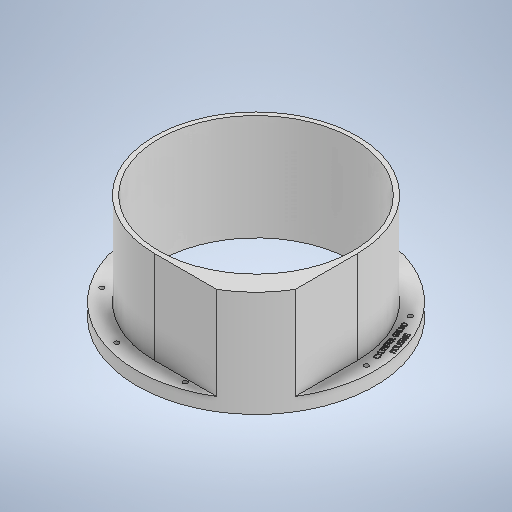
# Autodesk Inventor part: Cylinder Housing
Saved by Autodesk Inventor 2025 (Build 290162000, 162)
## iProperties
Created: 2025-06-17
Part Number: Cylinder Housing
Material: Generic
Document SubType Name: Modeling
Designer: mumin
Density: 1 g/cm^3
Appearance: Default
Author: mumin
Autodesk Inventor part; units mm, degrees
ref_plane "YZ Plane" through (0, 0, 0) normal (1, 0, 0) x (0, 1, 0)
ref_plane "XZ Plane" through (0, 0, 0) normal (0, 1, 0) x (-1, 0, 0)
ref_plane "XY Plane" through (0, 0, 0) normal (0, 0, 1) x (1, 0, 0)
sketch "Sketch1" plane through (0, 0, 0) normal (0, 1, 0) x (-1, 0, 0)
  circle A0 centre (0, 0) radius 110
  circle A1 centre (0, 0) radius 135
  dimension "d0" = 220
  dimension "d1" = 270
  constraints: 2 centre point, 2 coincident
  measures "d0" diameter of A0
  measures "d1" diameter of A1
extrude "Extrusion1" add sketch "Sketch1" along normal blind 15
sketch "Sketch5" plane through (0, 15, 0) normal (0, 1, 0) x (1, 0, 0)
  line L0 (-189, 0) -> (189, 0) projected
  point P0 (0, 0)
  point P1 (-125, 0)
  dimension "d23" = 125
  constraints: 1 point on line
  measures "d23" distance of point (0, 0) point (-125, 0)
hole "Hole2" at (-125, 15, 0) direction (0, -1, 0) diameter 5.2 end through all
pattern_circular "Circular Pattern1" count 10 over 360 about axis through (0, -10, 0) along (0, 1, 0) of "Hole2"
sketch "Sketch6" plane through (0, 0, 0) normal (0, 1, 0) x (-1, 0, 0)
  circle A0 centre (0, 0) radius 110 projected
  circle A1 centre (0, 0) radius 135 projected
  circle A2 centre (0, 0) radius 115
  line L0 (0, 115) -> (-115, 115)
  line L1 (-115, 115) -> (-115, 0)
  point P0 (-70.7107, 115)
  point P1 (-115, 70.7107)
  dimension "d27" = 230
  constraints: 4 end point, 2 point on circle, 2 tangent, 1 centre point, 1 coincident, 1 horizontal
  measures "d27" diameter of A2
extrude "Extrusion4" add sketch "Sketch6" along normal blind 120 contours L0 A2 L1 A1 | A2 picked at (-94.2438, 86.8114)
sketch "Sketch7" plane through (0, 15, 0) normal (0, 1, 0) x (1, 0, 0)
  line L0 (121.4652, 9.1206) -> (102.4195, 65.4859) construction
  line L1 (102.4195, 65.4859) -> (106.7219, 66.9397) construction
  line L2 (106.7219, 66.9397) -> (125.7676, 10.5743) construction
  line L3 (125.7676, 10.5743) -> (121.4652, 9.1206) construction
  spline S0 degree 2 poles (124.8327, 15.3814) (124.9884, 14.9208) (124.9407, 14.0365) (124.7258, 13.6474) knots 0 0 0 1 2 2 2
  spline S1 degree 2 poles (124.7258, 13.6474) (124.5147, 13.2596) (123.6985, 12.6373) (123.0996, 12.435) knots 0 0 0 1 2 2 2
  spline S2 degree 2 poles (123.0996, 12.435) (122.5046, 12.2339) (121.5193, 12.2389) (121.0957, 12.4165) knots 0 0 0 1 2 2 2
  spline S3 degree 2 poles (121.0957, 12.4165) (120.6811, 12.5929) (120.0852, 13.2555) (119.923, 13.7353) knots 0 0 0 1 2 2 2
  spline S4 degree 2 poles (119.923, 13.7353) (119.8426, 13.9733) (119.7703, 14.4151) (119.7644, 14.6098) knots 0 0 0 1 2 2 2
  spline S5 degree 2 poles (119.7644, 14.6098) (119.7624, 14.7802) (119.7968, 15.1468) (119.8281, 15.3327) knots 0 0 0 1 2 2 2
  line L4 (119.8281, 15.3327) -> (120.5881, 15.5895)
  line L5 (120.5881, 15.5895) -> (120.605, 15.5396)
  spline S6 degree 2 poles (120.605, 15.5396) (120.5567, 15.4293) (120.43, 15.0956) (120.3899, 14.8725) knots 0 0 0 1 2 2 2
  spline S7 degree 2 poles (120.3899, 14.8725) (120.351, 14.6583) (120.3683, 14.1894) (120.4617, 13.9131) knots 0 0 0 1 2 2 2
  spline S8 degree 2 poles (120.4617, 13.9131) (120.5642, 13.6098) (120.9966, 13.1529) (121.3033, 13.0298) knots 0 0 0 1 2 2 2
  spline S9 degree 2 poles (121.3033, 13.0298) (121.6126, 12.9119) (122.421, 12.937) (122.8778, 13.0914) knots 0 0 0 1 2 2 2
  spline S10 degree 2 poles (122.8778, 13.0914) (123.3653, 13.2561) (123.9887, 13.7276) (124.1618, 14.0128) knots 0 0 0 1 2 2 2
  spline S11 degree 2 poles (124.1618, 14.0128) (124.3285, 14.2915) (124.3862, 14.9055) (124.285, 15.2049) knots 0 0 0 1 2 2 2
  spline S12 degree 2 poles (124.285, 15.2049) (124.1929, 15.4775) (123.9016, 15.8966) (123.7409, 16.0433) knots 0 0 0 1 2 2 2
  spline S13 degree 2 poles (123.7409, 16.0433) (123.5827, 16.1823) (123.2885, 16.3694) (123.1909, 16.4177) knots 0 0 0 1 2 2 2
  line L6 (123.1909, 16.4177) -> (123.1754, 16.4638)
  line L7 (123.1754, 16.4638) -> (123.9277, 16.718)
  spline S14 degree 2 poles (123.9277, 16.718) (124.0539, 16.5853) (124.2816, 16.3543) (124.4092, 16.1793) knots 0 0 0 1 2 2 2
  spline S15 degree 2 poles (124.4092, 16.1793) (124.5483, 15.9953) (124.7367, 15.6655) (124.8327, 15.3814) knots 0 0 0 1 2 2 2
  line L8 (118.1942, 19.1303) -> (121.376, 18.4219)
  line L9 (121.376, 18.4219) -> (123.4719, 19.1301)
  line L10 (123.4719, 19.1301) -> (123.6847, 18.5006)
  line L11 (123.6847, 18.5006) -> (121.654, 17.8145)
  line L12 (121.654, 17.8145) -> (119.4887, 15.2993)
  line L13 (119.4887, 15.2993) -> (119.2526, 15.9979)
  line L14 (119.2526, 15.9979) -> (120.9232, 17.9268)
  line L15 (120.9232, 17.9268) -> (118.4199, 18.4623)
  line L16 (118.4199, 18.4623) -> (118.1942, 19.1303)
  line L17 (121.8558, 23.9131) -> (122.7832, 21.1685)
  line L18 (122.7832, 21.1685) -> (118.0463, 19.5679)
  line L19 (118.0463, 19.5679) -> (117.8336, 20.1974)
  line L20 (117.8336, 20.1974) -> (122.01, 21.6086)
  line L21 (122.01, 21.6086) -> (121.2954, 23.7237)
  line L22 (121.2954, 23.7237) -> (121.8558, 23.9131)
  line L23 (121.1307, 26.0589) -> (121.7507, 24.224)
  line L24 (121.7507, 24.224) -> (121.2671, 24.0606)
  line L25 (121.2671, 24.0606) -> (121.0634, 24.6633)
  line L26 (121.0634, 24.6633) -> (117.2939, 23.3895)
  line L27 (117.2939, 23.3895) -> (117.4975, 22.7869)
  line L28 (117.4975, 22.7869) -> (117.0138, 22.6234)
  line L29 (117.0138, 22.6234) -> (116.3938, 24.4583)
  line L30 (116.3938, 24.4583) -> (116.8775, 24.6217)
  line L31 (116.8775, 24.6217) -> (117.0812, 24.0191)
  line L32 (117.0812, 24.0191) -> (120.8507, 25.2928)
  line L33 (120.8507, 25.2928) -> (120.6471, 25.8955)
  line L34 (120.6471, 25.8955) -> (121.1307, 26.0589)
  line L35 (119.7221, 30.2277) -> (119.9608, 29.5214)
  line L36 (119.9608, 29.5214) -> (116.5847, 26.0454)
  line L37 (116.5847, 26.0454) -> (120.669, 27.4255)
  line L38 (120.669, 27.4255) -> (120.8674, 26.8381)
  line L39 (120.8674, 26.8381) -> (116.1305, 25.2376)
  line L40 (116.1305, 25.2376) -> (115.8283, 26.132)
  line L41 (115.8283, 26.132) -> (118.934, 29.307)
  line L42 (118.934, 29.307) -> (115.1837, 28.0398)
  line L43 (115.1837, 28.0398) -> (114.9852, 28.6271)
  line L44 (114.9852, 28.6271) -> (119.7221, 30.2277)
  spline S16 degree 2 poles (115.7712, 34.1233) (116.4199, 34.3425) (117.6417, 34.1695) (118.0826, 33.8266) knots 0 0 0 1 2 2 2
  spline S17 degree 2 poles (118.0826, 33.8266) (118.431, 33.5423) (118.8349, 32.8533) (119.0295, 32.2775) knots 0 0 0 1 2 2 2
  line L45 (119.0295, 32.2775) -> (119.3978, 31.1873)
  line L46 (119.3978, 31.1873) -> (114.661, 29.5867)
  line L47 (114.661, 29.5867) -> (114.2965, 30.6654)
  spline S18 degree 2 poles (114.2965, 30.6654) (114.0708, 31.3333) (114.0136, 32.1608) (114.0994, 32.4892) knots 0 0 0 1 2 2 2
  spline S19 degree 2 poles (114.0994, 32.4892) (114.2483, 33.0485) (115.0802, 33.8899) (115.7712, 34.1233) knots 0 0 0 1 2 2 2
  spline S20 degree 2 poles (115.9853, 33.4643) (115.4402, 33.2802) (114.7906, 32.6586) (114.6924, 32.2277) knots 0 0 0 1 2 2 2
  spline S21 degree 2 poles (114.6924, 32.2277) (114.6283, 31.9237) (114.6872, 31.3064) (114.8312, 30.8803) knots 0 0 0 1 2 2 2
  line L48 (114.8312, 30.8803) -> (114.9933, 30.4005)
  line L49 (114.9933, 30.4005) -> (118.64, 31.6327)
  line L50 (118.64, 31.6327) -> (118.4779, 32.1125)
  spline S22 degree 2 poles (118.4779, 32.1125) (118.3365, 32.5309) (117.9882, 33.1189) (117.7208, 33.3151) knots 0 0 0 1 2 2 2
  spline S23 degree 2 poles (117.7208, 33.3151) (117.3866, 33.57) (116.5381, 33.6511) (115.9853, 33.4643) knots 0 0 0 1 2 2 2
  line L51 (117.9049, 35.6056) -> (113.168, 34.005)
  line L52 (113.168, 34.005) -> (112.1667, 36.9685)
  line L53 (112.1667, 36.9685) -> (112.7271, 37.1578)
  line L54 (112.7271, 37.1578) -> (113.5158, 34.8239)
  line L55 (113.5158, 34.8239) -> (114.8132, 35.2623)
  line L56 (114.8132, 35.2623) -> (114.0778, 37.4389)
  line L57 (114.0778, 37.4389) -> (114.6382, 37.6282)
  line L58 (114.6382, 37.6282) -> (115.3737, 35.4517)
  line L59 (115.3737, 35.4517) -> (117.1318, 36.0458)
  line L60 (117.1318, 36.0458) -> (116.3431, 38.3797)
  line L61 (116.3431, 38.3797) -> (116.9036, 38.569)
  line L62 (116.9036, 38.569) -> (117.9049, 35.6056)
  line L63 (115.4314, 42.9259) -> (115.7077, 42.1083)
  line L64 (115.7077, 42.1083) -> (114.3288, 39.9743)
  line L65 (114.3288, 39.9743) -> (114.5726, 39.2527)
  line L66 (114.5726, 39.2527) -> (116.4574, 39.8895)
  line L67 (116.4574, 39.8895) -> (116.6701, 39.26)
  line L68 (116.6701, 39.26) -> (111.9332, 37.6594)
  line L69 (111.9332, 37.6594) -> (111.5207, 38.8801)
  spline S24 degree 2 poles (111.5207, 38.8801) (111.3833, 39.287) (111.2861, 39.8658) (111.363, 40.1698) knots 0 0 0 1 2 2 2
  spline S25 degree 2 poles (111.363, 40.1698) (111.4399, 40.4737) (111.8455, 40.9316) (112.2178, 41.0574) knots 0 0 0 1 2 2 2
  spline S26 degree 2 poles (112.2178, 41.0574) (112.736, 41.2325) (113.6175, 40.9401) (113.9395, 40.5442) knots 0 0 0 1 2 2 2
  line L70 (113.9395, 40.5442) -> (115.4314, 42.9259)
  spline S27 degree 2 poles (112.4895, 40.4178) (112.2822, 40.3478) (112.0129, 40.0943) (111.9612, 39.9057) knots 0 0 0 1 2 2 2
  spline S28 degree 2 poles (111.9612, 39.9057) (111.9183, 39.7415) (111.966, 39.3599) (112.0542, 39.0988) knots 0 0 0 1 2 2 2
  line L71 (112.0542, 39.0988) -> (112.2656, 38.4731)
  line L72 (112.2656, 38.4731) -> (114.0467, 39.075)
  line L73 (114.0467, 39.075) -> (113.8599, 39.6277)
  spline S29 degree 2 poles (113.8599, 39.6277) (113.7678, 39.9003) (113.5253, 40.3016) (113.325, 40.4008) knots 0 0 0 1 2 2 2
  spline S30 degree 2 poles (113.325, 40.4008) (113.1478, 40.4948) (112.7352, 40.5008) (112.4895, 40.4178) knots 0 0 0 1 2 2 2
  spline S31 degree 2 poles (114.0384, 47.3523) (114.2083, 46.8494) (114.1827, 45.9127) (113.9729, 45.5082) knots 0 0 0 1 2 2 2
  spline S32 degree 2 poles (113.9729, 45.5082) (113.7593, 45.1024) (112.938, 44.4699) (112.3354, 44.2663) knots 0 0 0 1 2 2 2
  spline S33 degree 2 poles (112.3354, 44.2663) (111.7634, 44.073) (110.7485, 44.0894) (110.3249, 44.2798) knots 0 0 0 1 2 2 2
  spline S34 degree 2 poles (110.3249, 44.2798) (109.9167, 44.4627) (109.2935, 45.193) (109.1236, 45.6959) knots 0 0 0 1 2 2 2
  spline S35 degree 2 poles (109.1236, 45.6959) (109.0419, 45.9377) (108.9631, 46.3987) (108.9571, 46.619) knots 0 0 0 1 2 2 2
  spline S36 degree 2 poles (108.9571, 46.619) (108.9487, 46.7958) (108.9853, 47.2444) (109.0065, 47.3842) knots 0 0 0 1 2 2 2
  line L74 (109.0065, 47.3842) -> (109.7666, 47.641)
  line L75 (109.7666, 47.641) -> (109.7847, 47.5873)
  spline S37 degree 2 poles (109.7847, 47.5873) (109.7213, 47.4332) (109.6175, 47.1202) (109.5878, 46.8535) knots 0 0 0 1 2 2 2
  spline S38 degree 2 poles (109.5878, 46.8535) (109.5567, 46.6292) (109.5974, 46.0912) (109.6934, 45.8071) knots 0 0 0 1 2 2 2
  spline S39 degree 2 poles (109.6934, 45.8071) (109.9242, 45.1239) (111.2383, 44.627) (112.0944, 44.9162) knots 0 0 0 1 2 2 2
  spline S40 degree 2 poles (112.0944, 44.9162) (112.5704, 45.077) (113.2091, 45.5409) (113.3834, 45.8351) knots 0 0 0 1 2 2 2
  spline S41 degree 2 poles (113.3834, 45.8351) (113.5604, 46.1215) (113.623, 46.7842) (113.5011, 47.1451) knots 0 0 0 1 2 2 2
  spline S42 degree 2 poles (113.5011, 47.1451) (113.4116, 47.4099) (113.1558, 47.9137) (113.0181, 48.0682) knots 0 0 0 1 2 2 2
  line L76 (113.0181, 48.0682) -> (111.7936, 47.6544)
  line L77 (111.7936, 47.6544) -> (112.1645, 46.5566)
  line L78 (112.1645, 46.5566) -> (111.6117, 46.3698)
  line L79 (111.6117, 46.3698) -> (111.0307, 48.0895)
  line L80 (111.0307, 48.0895) -> (113.0997, 48.7886)
  spline S43 degree 2 poles (113.0997, 48.7886) (113.1936, 48.6878) (113.4962, 48.3367) (113.6045, 48.1808) knots 0 0 0 1 2 2 2
  spline S44 degree 2 poles (113.6045, 48.1808) (113.7527, 47.97) (113.9489, 47.6172) (114.0384, 47.3523) knots 0 0 0 1 2 2 2
  line L81 (113.3198, 49.1752) -> (108.0433, 49.1715)
  line L82 (108.0433, 49.1715) -> (107.7813, 49.9469)
  line L83 (107.7813, 49.9469) -> (111.9786, 53.1444)
  line L84 (111.9786, 53.1444) -> (112.203, 52.4803)
  line L85 (112.203, 52.4803) -> (111.0239, 51.6029)
  line L86 (111.0239, 51.6029) -> (111.6349, 49.7949)
  line L87 (111.6349, 49.7949) -> (113.1045, 49.8124)
  line L88 (113.1045, 49.8124) -> (113.3198, 49.1752)
  line L89 (110.5449, 51.2486) -> (108.5624, 49.7618)
  line L90 (108.5624, 49.7618) -> (111.0391, 49.786)
  line L91 (111.0391, 49.786) -> (110.5449, 51.2486)
  line L92 (110.8994, 56.3381) -> (111.8268, 53.5935)
  line L93 (111.8268, 53.5935) -> (107.09, 51.9929)
  line L94 (107.09, 51.9929) -> (106.8772, 52.6225)
  line L95 (106.8772, 52.6225) -> (111.0537, 54.0337)
  line L96 (111.0537, 54.0337) -> (110.339, 56.1488)
  line L97 (110.339, 56.1488) -> (110.8994, 56.3381)
  line L98 (104.8344, 58.6683) -> (110.1225, 58.6375)
  line L99 (110.1225, 58.6375) -> (110.3521, 57.9581)
  line L100 (110.3521, 57.9581) -> (106.1664, 54.726)
  line L101 (106.1664, 54.726) -> (105.9382, 55.4016)
  line L102 (105.9382, 55.4016) -> (109.4292, 58.044)
  line L103 (109.4292, 58.044) -> (105.051, 58.0273)
  line L104 (105.051, 58.0273) -> (104.8344, 58.6683)
  spline S45 degree 2 poles (104.0902, 62.6553) (104.3142, 63.0304) (105.1343, 63.6411) (105.7254, 63.8408) knots 0 0 0 1 2 2 2
  spline S46 degree 2 poles (105.7254, 63.8408) (106.3012, 64.0354) (107.3326, 64.0589) (107.7408, 63.8888) knots 0 0 0 1 2 2 2
  spline S47 degree 2 poles (107.7408, 63.8888) (108.1695, 63.7086) (108.7449, 63.0434) (108.9019, 62.579) knots 0 0 0 1 2 2 2
  spline S48 degree 2 poles (108.9019, 62.579) (109.064, 62.0991) (108.9971, 61.2211) (108.7732, 60.8333) knots 0 0 0 1 2 2 2
  spline S49 degree 2 poles (108.7732, 60.8333) (108.5505, 60.4544) (107.724, 59.85) (107.1405, 59.6529) knots 0 0 0 1 2 2 2
  spline S50 degree 2 poles (107.1405, 59.6529) (106.5455, 59.4518) (105.5398, 59.4413) (105.1214, 59.6036) knots 0 0 0 1 2 2 2
  spline S51 degree 2 poles (105.1214, 59.6036) (104.7132, 59.7736) (104.1262, 60.4349) (103.9654, 60.9109) knots 0 0 0 1 2 2 2
  spline S52 degree 2 poles (103.9654, 60.9109) (103.802, 61.3946) (103.8777, 62.2841) (104.0902, 62.6553) knots 0 0 0 1 2 2 2
  spline S53 degree 2 poles (105.9472, 63.1844) (105.4789, 63.0262) (104.8222, 62.5776) (104.6464, 62.3129) knots 0 0 0 1 2 2 2
  spline S54 degree 2 poles (104.6464, 62.3129) (104.4643, 62.0418) (104.3976, 61.4291) (104.5092, 61.099) knots 0 0 0 1 2 2 2
  spline S55 degree 2 poles (104.5092, 61.099) (104.6246, 60.7573) (105.0364, 60.3234) (105.3559, 60.2132) knots 0 0 0 1 2 2 2
  spline S56 degree 2 poles (105.3559, 60.2132) (105.6613, 60.1068) (106.4581, 60.1536) (106.9187, 60.3093) knots 0 0 0 1 2 2 2
  spline S57 degree 2 poles (106.9187, 60.3093) (107.8515, 60.6245) (108.5773, 61.7422) (108.3555, 62.3986) knots 0 0 0 1 2 2 2
  spline S58 degree 2 poles (108.3555, 62.3986) (108.1337, 63.055) (106.88, 63.4996) (105.9472, 63.1844) knots 0 0 0 1 2 2 2
  line L105 (127.9908, 31.4734) -> (128.2035, 30.8439)
  line L106 (128.2035, 30.8439) -> (125.885, 30.0604)
  line L107 (125.885, 30.0604) -> (126.6217, 27.8801)
  line L108 (126.6217, 27.8801) -> (128.9403, 28.6635)
  line L109 (128.9403, 28.6635) -> (129.153, 28.034)
  line L110 (129.153, 28.034) -> (124.4161, 26.4334)
  line L111 (124.4161, 26.4334) -> (124.2034, 27.0629)
  line L112 (124.2034, 27.0629) -> (126.0613, 27.6907)
  line L113 (126.0613, 27.6907) -> (125.3246, 29.8711)
  line L114 (125.3246, 29.8711) -> (123.4666, 29.2433)
  line L115 (123.4666, 29.2433) -> (123.2539, 29.8728)
  line L116 (123.2539, 29.8728) -> (127.9908, 31.4734)
  spline S59 degree 2 poles (122.3386, 34.3665) (122.5625, 34.7416) (123.3826, 35.3523) (123.9738, 35.552) knots 0 0 0 1 2 2 2
  spline S60 degree 2 poles (123.9738, 35.552) (124.5496, 35.7466) (125.581, 35.77) (125.9891, 35.6) knots 0 0 0 1 2 2 2
  spline S61 degree 2 poles (125.9891, 35.6) (126.4178, 35.4198) (126.9933, 34.7546) (127.1502, 34.2901) knots 0 0 0 1 2 2 2
  spline S62 degree 2 poles (127.1502, 34.2901) (127.3124, 33.8103) (127.2455, 32.9323) (127.0216, 32.5445) knots 0 0 0 1 2 2 2
  spline S63 degree 2 poles (127.0216, 32.5445) (126.7989, 32.1656) (125.9724, 31.5612) (125.3889, 31.3641) knots 0 0 0 1 2 2 2
  spline S64 degree 2 poles (125.3889, 31.3641) (124.7939, 31.163) (123.7881, 31.1525) (123.3697, 31.3148) knots 0 0 0 1 2 2 2
  spline S65 degree 2 poles (123.3697, 31.3148) (122.9616, 31.4848) (122.3746, 32.1461) (122.2137, 32.6221) knots 0 0 0 1 2 2 2
  spline S66 degree 2 poles (122.2137, 32.6221) (122.0503, 33.1058) (122.1261, 33.9953) (122.3386, 34.3665) knots 0 0 0 1 2 2 2
  spline S67 degree 2 poles (124.1956, 34.8956) (123.7273, 34.7374) (123.0705, 34.2888) (122.8948, 34.0241) knots 0 0 0 1 2 2 2
  spline S68 degree 2 poles (122.8948, 34.0241) (122.7127, 33.753) (122.646, 33.1403) (122.7575, 32.8101) knots 0 0 0 1 2 2 2
  spline S69 degree 2 poles (122.7575, 32.8101) (122.873, 32.4685) (123.2848, 32.0345) (123.6043, 31.9244) knots 0 0 0 1 2 2 2
  spline S70 degree 2 poles (123.6043, 31.9244) (123.9097, 31.818) (124.7065, 31.8648) (125.1671, 32.0205) knots 0 0 0 1 2 2 2
  spline S71 degree 2 poles (125.1671, 32.0205) (126.0999, 32.3357) (126.8257, 33.4534) (126.6039, 34.1098) knots 0 0 0 1 2 2 2
  spline S72 degree 2 poles (126.6039, 34.1098) (126.3821, 34.7662) (125.1284, 35.2108) (124.1956, 34.8956) knots 0 0 0 1 2 2 2
  spline S73 degree 2 poles (125.6495, 38.7315) (125.7909, 38.313) (125.7822, 37.6173) (125.6374, 37.3245) knots 0 0 0 1 2 2 2
  spline S74 degree 2 poles (125.6374, 37.3245) (125.476, 36.992) (124.8538, 36.5551) (124.3471, 36.3839) knots 0 0 0 1 2 2 2
  line L117 (124.3471, 36.3839) -> (121.3913, 35.3851)
  line L118 (121.3913, 35.3851) -> (121.1786, 36.0147)
  line L119 (121.1786, 36.0147) -> (124.1344, 37.0134)
  spline S75 degree 2 poles (124.1344, 37.0134) (124.4645, 37.1249) (124.8812, 37.3599) (125.0215, 37.5398) knots 0 0 0 1 2 2 2
  spline S76 degree 2 poles (125.0215, 37.5398) (125.1706, 37.7313) (125.2185, 38.2351) (125.1121, 38.5499) knots 0 0 0 1 2 2 2
  spline S77 degree 2 poles (125.1121, 38.5499) (125.0123, 38.8454) (124.6608, 39.2399) (124.4261, 39.3018) knots 0 0 0 1 2 2 2
  spline S78 degree 2 poles (124.4261, 39.3018) (124.2055, 39.3598) (123.7355, 39.2951) (123.4169, 39.1874) knots 0 0 0 1 2 2 2
  line L120 (123.4169, 39.1874) -> (120.4458, 38.1835)
  line L121 (120.4458, 38.1835) -> (120.2331, 38.813)
  line L122 (120.2331, 38.813) -> (123.1888, 39.8118)
  spline S79 degree 2 poles (123.1888, 39.8118) (123.684, 39.9791) (124.4578, 40.0181) (124.7852, 39.8465) knots 0 0 0 1 2 2 2
  spline S80 degree 2 poles (124.7852, 39.8465) (125.0844, 39.6953) (125.5017, 39.1691) (125.6495, 38.7315) knots 0 0 0 1 2 2 2
  spline S81 degree 2 poles (124.3034, 42.6647) (124.4772, 42.1503) (124.5061, 41.356) (124.4602, 40.9856) knots 0 0 0 1 2 2 2
  line L123 (124.4602, 40.9856) -> (123.6694, 40.7184)
  line L124 (123.6694, 40.7184) -> (123.6539, 40.7644)
  spline S82 degree 2 poles (123.6539, 40.7644) (123.8405, 41.1739) (123.8971, 42.0698) (123.7739, 42.4345) knots 0 0 0 1 2 2 2
  spline S83 degree 2 poles (123.7739, 42.4345) (123.5975, 42.9565) (122.9834, 43.3435) (122.6264, 43.2229) knots 0 0 0 1 2 2 2
  spline S84 degree 2 poles (122.6264, 43.2229) (122.3423, 43.1269) (122.0839, 42.7274) (122.0981, 42.3943) knots 0 0 0 1 2 2 2
  spline S85 degree 2 poles (122.0981, 42.3943) (122.1106, 42.1547) (122.1493, 41.7615) (122.1723, 41.4656) knots 0 0 0 1 2 2 2
  spline S86 degree 2 poles (122.1723, 41.4656) (122.1901, 41.1979) (122.1253, 40.7441) (122.0185, 40.5412) knots 0 0 0 1 2 2 2
  spline S87 degree 2 poles (122.0185, 40.5412) (121.9104, 40.3421) (121.5427, 40.0382) (121.2663, 39.9448) knots 0 0 0 1 2 2 2
  spline S88 degree 2 poles (121.2663, 39.9448) (120.6905, 39.7503) (119.6077, 40.3852) (119.373, 41.08) knots 0 0 0 1 2 2 2
  spline S89 degree 2 poles (119.373, 41.08) (119.2381, 41.4792) (119.1568, 42.2387) (119.204, 42.5925) knots 0 0 0 1 2 2 2
  line L125 (119.204, 42.5925) -> (119.9564, 42.8468)
  line L126 (119.9564, 42.8468) -> (119.972, 42.8007)
  spline S90 degree 2 poles (119.972, 42.8007) (119.8412, 42.5042) (119.7728, 41.6941) (119.9038, 41.3064) knots 0 0 0 1 2 2 2
  spline S91 degree 2 poles (119.9038, 41.3064) (120.0516, 40.8688) (120.6453, 40.4663) (120.9792, 40.5792) knots 0 0 0 1 2 2 2
  spline S92 degree 2 poles (120.9792, 40.5792) (121.2786, 40.6804) (121.528, 41.1196) (121.5074, 41.4462) knots 0 0 0 1 2 2 2
  spline S93 degree 2 poles (121.5074, 41.4462) (121.4937, 41.664) (121.436, 42.2903) (121.4288, 42.5017) knots 0 0 0 1 2 2 2
  spline S94 degree 2 poles (121.4288, 42.5017) (121.4137, 43.0398) (121.8634, 43.6964) (122.3048, 43.8456) knots 0 0 0 1 2 2 2
  spline S95 degree 2 poles (122.3048, 43.8456) (122.585, 43.9403) (123.199, 43.8954) (123.4558, 43.7555) knots 0 0 0 1 2 2 2
  spline S96 degree 2 poles (123.4558, 43.7555) (123.7396, 43.5991) (124.1568, 43.0985) (124.3034, 42.6647) knots 0 0 0 1 2 2 2
  line L127 (122.8817, 46.5938) -> (123.5017, 44.759)
  line L128 (123.5017, 44.759) -> (123.018, 44.5955)
  line L129 (123.018, 44.5955) -> (122.8143, 45.1982)
  line L130 (122.8143, 45.1982) -> (119.0448, 43.9245)
  line L131 (119.0448, 43.9245) -> (119.2484, 43.3218)
  line L132 (119.2484, 43.3218) -> (118.7648, 43.1584)
  line L133 (118.7648, 43.1584) -> (118.1448, 44.9932)
  line L134 (118.1448, 44.9932) -> (118.6284, 45.1567)
  line L135 (118.6284, 45.1567) -> (118.8321, 44.554)
  line L136 (118.8321, 44.554) -> (122.6016, 45.8277)
  line L137 (122.6016, 45.8277) -> (122.398, 46.4304)
  line L138 (122.398, 46.4304) -> (122.8817, 46.5938)
  line L139 (121.473, 50.7626) -> (121.7117, 50.0563)
  line L140 (121.7117, 50.0563) -> (118.3356, 46.5803)
  line L141 (118.3356, 46.5803) -> (122.4199, 47.9604)
  line L142 (122.4199, 47.9604) -> (122.6184, 47.3731)
  line L143 (122.6184, 47.3731) -> (117.8815, 45.7725)
  line L144 (117.8815, 45.7725) -> (117.5792, 46.6669)
  line L145 (117.5792, 46.6669) -> (120.685, 49.8419)
  line L146 (120.685, 49.8419) -> (116.9346, 48.5747)
  line L147 (116.9346, 48.5747) -> (116.7361, 49.162)
  line L148 (116.7361, 49.162) -> (121.473, 50.7626)
  spline S97 degree 2 poles (120.5703, 53.738) (120.7402, 53.2351) (120.7146, 52.2984) (120.5048, 51.8939) knots 0 0 0 1 2 2 2
  spline S98 degree 2 poles (120.5048, 51.8939) (120.2912, 51.4881) (119.4699, 50.8556) (118.8673, 50.652) knots 0 0 0 1 2 2 2
  spline S99 degree 2 poles (118.8673, 50.652) (118.2953, 50.4587) (117.2804, 50.475) (116.8568, 50.6655) knots 0 0 0 1 2 2 2
  spline S100 degree 2 poles (116.8568, 50.6655) (116.4486, 50.8483) (115.8255, 51.5787) (115.6555, 52.0816) knots 0 0 0 1 2 2 2
  spline S101 degree 2 poles (115.6555, 52.0816) (115.5738, 52.3234) (115.4951, 52.7843) (115.489, 53.0047) knots 0 0 0 1 2 2 2
  spline S102 degree 2 poles (115.489, 53.0047) (115.4806, 53.1815) (115.5172, 53.6301) (115.5384, 53.7699) knots 0 0 0 1 2 2 2
  line L149 (115.5384, 53.7699) -> (116.2985, 54.0267)
  line L150 (116.2985, 54.0267) -> (116.3166, 53.9729)
  spline S103 degree 2 poles (116.3166, 53.9729) (116.2532, 53.8189) (116.1494, 53.5059) (116.1198, 53.2392) knots 0 0 0 1 2 2 2
  spline S104 degree 2 poles (116.1198, 53.2392) (116.0887, 53.0149) (116.1293, 52.4769) (116.2253, 52.1928) knots 0 0 0 1 2 2 2
  spline S105 degree 2 poles (116.2253, 52.1928) (116.4562, 51.5095) (117.7703, 51.0126) (118.6263, 51.3019) knots 0 0 0 1 2 2 2
  spline S106 degree 2 poles (118.6263, 51.3019) (119.1023, 51.4627) (119.741, 51.9266) (119.9154, 52.2208) knots 0 0 0 1 2 2 2
  spline S107 degree 2 poles (119.9154, 52.2208) (120.0923, 52.5072) (120.1549, 53.1699) (120.033, 53.5308) knots 0 0 0 1 2 2 2
  spline S108 degree 2 poles (120.033, 53.5308) (119.9435, 53.7956) (119.6877, 54.2994) (119.55, 54.4539) knots 0 0 0 1 2 2 2
  line L151 (119.55, 54.4539) -> (118.3255, 54.0401)
  line L152 (118.3255, 54.0401) -> (118.6964, 52.9423)
  line L153 (118.6964, 52.9423) -> (118.1437, 52.7555)
  line L154 (118.1437, 52.7555) -> (117.5626, 54.4752)
  line L155 (117.5626, 54.4752) -> (119.6316, 55.1743)
  spline S109 degree 2 poles (119.6316, 55.1743) (119.7256, 55.0735) (120.0281, 54.7224) (120.1364, 54.5665) knots 0 0 0 1 2 2 2
  spline S110 degree 2 poles (120.1364, 54.5665) (120.2846, 54.3557) (120.4808, 54.0028) (120.5703, 53.738) knots 0 0 0 1 2 2 2
  point P0 (0, 0)
  constraints: 2 other
emboss "Emboss1" sketch "Sketch7" operation cut depth 1 direction (0, -1, 0)
body "Solid1"
